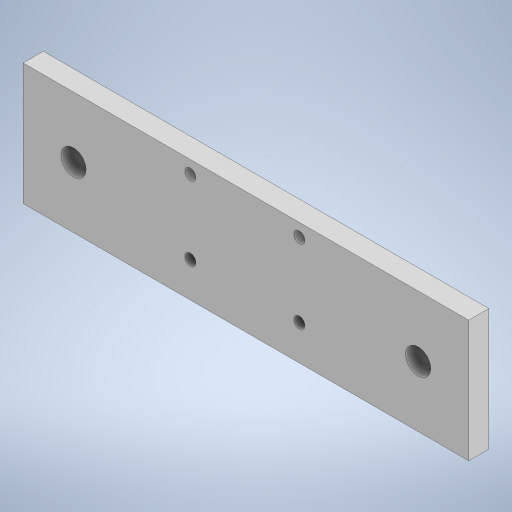
# Autodesk Inventor part: A4988_driver_holder
Saved by Autodesk Inventor 2024 (Build 280153000, 153)
## iProperties
Created: 2026-01-01
Part Number: A4988_driver_holder
Material: Generic
Document SubType Name: Modeling
Designer: schar
Density: 1 g/cm^3
Appearance: Default
Author: schar
Autodesk Inventor part; units mm, degrees
ref_plane "YZ Plane" through (0, 0, 0) normal (1, 0, 0) x (0, 1, 0)
ref_plane "Work Plane1" through (24.13, 24.13, 0) normal (0, 0, -1) x (-1, 0, 0)
sketch "Sketch1" plane through (24.13, 24.13, 0) normal (0, 0, -1) x (-1, 0, 0)
  line L0 (0, 0) -> (21.59, 0) projected
  line L1 (-2.54, -21.59) -> (-2.54, -2.54) projected
  line L2 (-2.54, -2.54) -> (-2.54, 0)
  line L3 (-2.54, 0) -> (0, 0)
  line L4 (24.13, -24.13) -> (-2.54, -24.13)
  line L5 (-2.54, -24.13) -> (-2.54, 0)
  line L6 (-2.54, 0) -> (24.13, 0)
  line L7 (24.13, 0) -> (24.13, -24.13)
  line L8 (10.795, -24.13) -> (10.414, 0)
  line L9 (24.13, -12.065) -> (10.6045, -12.065)
  line L10 (-33.5455, 0) -> (54.7545, 0)
  line L11 (54.7545, 0) -> (54.7545, -24.13)
  line L12 (54.7545, -24.13) -> (-33.5455, -24.13)
  line L13 (-33.5455, -24.13) -> (-33.5455, 0)
  line L14 (-33.5455, 0) -> (54.7545, -24.13) construction
  line L15 (54.7545, 0) -> (-33.5455, -24.13) construction
  dimension "d1" = 88.3
  constraints: 28 end point, 5 midpoint, 4 parallel, 3 perpendicular, 2 horizontal, 1 point on line, 1 vertical
  measures "d1" distance of L11.end L12.end
extrude "Extrusion1" add sketch "Sketch1" along normal blind 4
sketch "Sketch2" plane through (24.13, 24.13, 0) normal (0, 0, 1) x (1, 0, 0)
  circle A0 centre (-21.59, -17.145) radius 1.1 projected
  circle A1 centre (-21.59, -17.145) radius 1.1
  circle A2 centre (0, -17.145) radius 1.1 projected
  circle A3 centre (0, -17.145) radius 1.1
  circle A4 centre (0, -2.54) radius 1.1 projected
  circle A5 centre (0, -2.54) radius 1.1
  circle A6 centre (-21.59, -2.54) radius 1.1 projected
  circle A7 centre (-21.59, -2.54) radius 1.1
  point P0 (-24.13, -24.13)
  constraints: 4 centre point, 4 coincident
extrude "Extrusion2" cut sketch "Sketch2" against normal blind 4
ref_plane "Work Plane2" through (24.13, 24.13, 0) normal (0, 0, 1) x (1, 0, 0)
sketch "Sketch3" plane through (24.13, 24.13, 0) normal (0, 0, 1) x (1, 0, 0)
  line L0 (-54.7545, -24.13) -> (-54.7545, 0) projected
  line L1 (-54.7545, -12.065) -> (-44.7545, -12.065)
  line L2 (33.5455, 0) -> (33.5455, -24.13) projected
  line L3 (33.5455, -12.065) -> (23.5455, -12.065)
  circle A0 centre (-44.7545, -12.065) radius 2.5
  circle A1 centre (23.5455, -12.065) radius 2.5
  point P0 (-24.13, -24.13)
  dimension "d6" = 10
  dimension "d7" = 10
  dimension "d8" = 5
  dimension "d9" = 5
  constraints: 4 end point, 2 centre point, 2 coincident, 2 horizontal, 2 midpoint
  measures "d6" distance of L1.start L1.end
  measures "d7" distance of L3.start L3.end
  measures "d8" diameter of A0
  measures "d9" diameter of A1
extrude "Extrusion3" cut sketch "Sketch3" against normal blind 4
body "Solid1"
